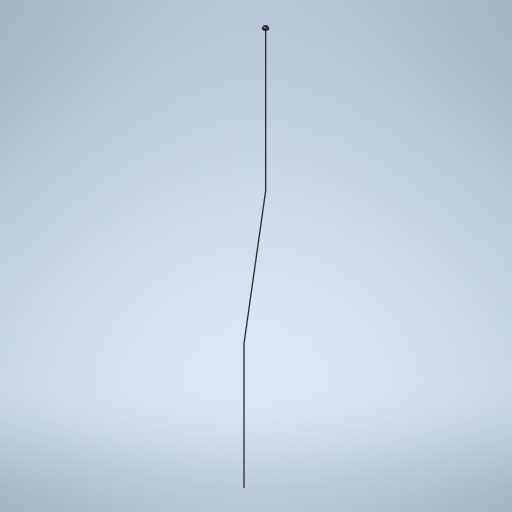
# Autodesk Inventor part: cable anular
Saved by Autodesk Inventor 2023 (Build 270158000, 158)
## iProperties
Created: 2022-10-27
Part Number: cable anular
Material: Generic
Document SubType Name: Modeling
Designer: Xiaba
Density: 1 g/cm^3
Appearance: Default
Author: Xiaba
Autodesk Inventor part; units mm, degrees
ref_plane "YZ Plane" through (0, 0, 0) normal (1, 0, 0) x (0, 1, 0)
ref_plane "XZ Plane" through (0, 0, 0) normal (0, 1, 0) x (-1, 0, 0)
sketch "Sketch1" plane through (0, 0, 0) normal (0, 1, 0) x (-1, 0, 0)
  circle A0 centre (0, 0) radius 0.25
  dimension "d0" = 0.5
  constraints: 1 centre point, 1 coincident
  measures "d0" diameter of A0
sketch "Sketch2" plane through (0, 0, 0) normal (1, 0, 0) x (0, 1, 0)
  line L0 (0, 0) -> (66.843, 0)
  line L1 (66.843, 0) -> (131.0178, -11.4428)
  line L2 (131.0178, -11.4428) -> (206.1678, -11.4428)
  dimension "d1" = 66.843
  dimension "d2" = 169.89
  dimension "d3" = 65.187
  dimension "d4" = 75.15
  constraints: 6 end point, 2 horizontal
  measures "d1" distance of L0.start L0.end
  measures "d2" angle of L0 L1
  measures "d3" distance of L0.end L1.end
  measures "d4" distance of L1.end L2.end
sweep "Sweep1" add profiles "Sketch1" path "Sketch2"
sketch "Sketch3" plane through (0, 206.1678, -11.4428) normal (0, 1, 0) x (1, 0, 0)
  line L0 (0, 0) -> (-0.3702, 0) construction
  point P0 (0, -11.4428)
  constraints: 2 end point, 1 horizontal
ref_plane "Work Plane1" through (0, 206.1678, -11.4428) normal (0, 0, -1) x (-1, 0, 0)
sketch "Sketch4" plane through (0, 206.1678, -11.4428) normal (0, 0, -1) x (-1, 0, 0)
  line L0 (0.25, 0) -> (-0.25, 0) projected
  circle A0 centre (0, 0) radius 1.5
  line L1 (0, 1.5) -> (0, 0)
  line L2 (0, 0) -> (-1.5, 0)
  point P0 (0, -206.1678)
  dimension "d8" = 3
  constraints: 4 end point, 2 point on circle, 1 centre point, 1 midpoint, 1 perpendicular, 1 vertical
  measures "d8" diameter of A0
revolve "Revolution1" add sketch "Sketch4" angle 360 about axis through (0, 207.6678, -11.4428) along (0, -1, 0) picked at (-0.1113, 0.9875) contours L0 L2 A0 L1
fillet "Fillet1" radius 0.2 1 edges at (-1.5, 206.1678, -11.4428)
sketch "Sketch5" plane through (0, 0, 0) normal (0, -1, 0) x (1, 0, 0)
  circle A0 centre (0, 0) radius 0.25 projected
extrude "Extrusion1" add sketch "Sketch5" along normal blind 0.1
body "Solid1"
